Autodesk Fusion 360 part; units mm, degrees
(part 2 of 2)
sketch "Sketch1" plane through (0, 0, 8.8) normal (0, 0, 1) x (-1, 0, 0) in component "label"
  circle A0 centre (-21, -32) radius 7.5
  arc A1 (-30.8, -38) -> (-28, -40.8) centre (-28, -38) ccw
  line L0 (-28, -40.8) -> (-1, -40.8)
  arc A2 (-1, -40.8) -> (1.8, -37.997) centre (-1, -38) ccw
  line L1 (1.8, -37.997) -> (1.8, -1)
  arc A3 (1.8, -1) -> (-1, 1.8) centre (-1, -1) ccw
  line L2 (-1, 1.8) -> (-28, 1.8)
  arc A4 (-28, 1.8) -> (-30.8, -1) centre (-28, -1) ccw
  line L3 (-30.8, -1) -> (-30.8, -38)
  line L4 (-1, -40.8) -> (-28, -40.8)
  arc A5 (-1, -40.8) -> (1.8, -37.997) centre (-1, -38) ccw
  line L5 (1.8, -1) -> (1.8, -37.997)
  arc A6 (1.8, -1) -> (-1, 1.8) centre (-1, -1) ccw
  line L6 (-28, 1.8) -> (-1, 1.8)
  arc A7 (-28, 1.8) -> (-30.8, -1) centre (-28, -1) ccw
  line L7 (-30.8, -38) -> (-30.8, -1)
  arc A8 (-30.8, -38) -> (-28, -40.8) centre (-28, -38) ccw
  circle A9 centre (-21, -32) radius 7.5
  circle A10 centre (-7, -32) radius 4.5 construction
  circle A11 centre (-7, -18) radius 4.5 construction
  circle A12 centre (-21, -18) radius 4.5 construction
  circle A13 centre (-7, -32) radius 5
  circle A14 centre (-7, -18) radius 5
  circle A15 centre (-21, -18) radius 5
  dimension "d268" = 0.5
  dimension "d269" = 0.5
  dimension "d270" = 0.5
extrude "Extrude1'''" add sketch "Sketch1" along normal blind 0.1 separate body makes body 7 in component "label"
component "PCB" placed x (1, 0, 0) y (0, 1, 0) z (0, 0, 1) at (0, 0, 0)
component "bottom shell" placed x (1, 0, 0) y (0, 1, 0) z (0, 0, 1) at (0, 0, 0)
component "top shell" placed x (1, 0, 0) y (0, 1, 0) z (0, 0, 1) at (0, 0, 0)
component "label" placed x (1, 0, 0) y (0, 1, 0) z (0, 0, 1) at (0, 0, 0)
equation "d28 = tol"
equation "tol = 0.3 mm"
equation "wall = 2.5 mm"
equation "d33 = wall"
equation "pad_depression = 1.5 mm"
equation "d51 = -pad_depression"
equation "bottom_height = 8 mm"
equation "overlap = 1.5 mm"
equation "d55 = -bottom_height + overlap"
equation "d57 = -bottom_height"
equation "d64 = wall * 0.4"
equation "pin_width = 8 mm"
equation "pin_thickness = 2.5 mm"
equation "pin_length = 6 mm"
equation "d69 = pin_thickness"
equation "d70 = pin_width"
equation "d72 = pin_width"
equation "d73 = pin_thickness"
equation "d75 = pin_width * 0.6"
equation "d76 = pin_thickness"
equation "d78 = pin_thickness"
equation "d79 = pin_width"
equation "stem_height = bottom_height - 2 mm"
equation "d85 = wall"
equation "d87 = -overlap"
equation "d89 = -stem_height"
equation "d91 = -pin_length"
equation "hook_height = 2.7 mm"
equation "hook_depth = 0.8 mm"
equation "d95 = hook_depth"
equation "d96 = hook_height"
equation "d97 = hook_depth"
equation "d98 = hook_height"
equation "d99 = hook_height"
equation "d100 = hook_depth"
equation "d101 = hook_height"
equation "d102 = hook_depth"
equation "d103 = -pin_width * 0.6"
equation "d105 = -pin_width"
equation "d107 = -pin_width"
equation "d109 = -pin_width"
equation "d113 = tol"
equation "d114 = tol"
equation "d115 = tol"
equation "d116 = tol"
equation "d117 = tol"
equation "d118 = tol"
equation "d119 = tol"
equation "d120 = tol"
equation "d121 = tol"
equation "d122 = tol"
equation "d123 = tol"
equation "d124 = tol"
equation "d125 = tol"
equation "d126 = tol"
equation "d127 = tol"
equation "d128 = tol"
equation "hook_depression_top = 0.2 mm"
equation "hook_depression_bottom = hook_depth + 0.2 mm"
equation "d131 = -hook_depression_bottom"
equation "d133 = -hook_depression_top"
equation "d135 = -hook_depression_bottom"
equation "d137 = -hook_depression_top"
equation "d139 = -hook_depression_bottom"
equation "d141 = -hook_depression_top"
equation "d143 = -hook_depression_bottom"
equation "d145 = -hook_depression_top"
equation "tol_rad = 0.5 mm"
equation "d177 = tol"
equation "d178 = tol"
equation "d179 = tol"
equation "d180 = tol"
equation "d182 = wall + tol"
equation "d183 = wall + tol"
equation "d189 = tol + 0.6 * wall"
equation "d190 = d189"
equation "d191 = d189"
equation "d192 = d189"
equation "d193 = d189"
equation "d194 = d189"
equation "d195 = d189"
equation "d198 = d182"
equation "d199 = d182"
equation "d200 = 0.50 mm"
equation "d215 = d200"
equation "d216 = d200"
equation "d217 = d200"
equation "d218 = d200"
equation "d219 = d200"
equation "d220 = d200"
equation "d237 = tol"
equation "d238 = tol"
equation "d239 = tol"
equation "d240 = tol"
equation "d241 = tol"
equation "d242 = tol"
equation "d243 = tol"
equation "d244 = tol"
equation "d245 = tol"
equation "RCAdia = 9.0 mm"
equation "d265 = RCAdia"
equation "d266 = RCAdia"
equation "d267 = RCAdia"
equation "d269 = d268"
equation "d270 = d268"
named bodies: "PCB", "label"
